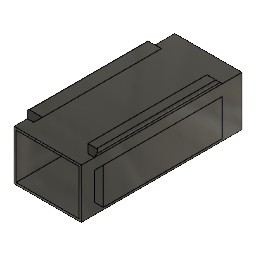
Res_Box v9 (Autodesk Fusion 360 design; units mm, degrees)
Autodesk Fusion 360 part; units mm, degrees
sketch "Boceto1" plane through (0, 0, 0) normal (0, 1, 0) x (1, 0, 0)
  line L0 (0, -22.6) -> (30.6, -22.6)
  line L1 (30.6, -22.6) -> (30.6, 0)
  line L2 (30.6, 0) -> (0, 0)
  line L3 (0, 0) -> (0, -22.6)
  dimension "d1" = 22.6
  dimension "d2" = 30.6
  constraint horizontal L0
  constraint vertical L1
  constraint horizontal L2
  constraint vertical L3
  constraint coincident L2.end L3.start
  measures "d1" distance of L0.end L1.end
  measures "d2" distance of L0.start L0.end
extrude "Extruir1" add sketch "Boceto1" along normal blind 73
shell "Vaciado1" thickness 1 removed faces 1 at (20.4, 0, 15.0667)
sketch "Boceto2" plane through (0, 0, 0) normal (0, -1, 0) x (1, 0, 0)
  line L0 (0, 22.6) -> (0, 0)
  line L1 (0, 0) -> (30.6, 0)
  line L2 (30.6, 0) -> (30.6, 22.6)
  line L3 (30.6, 22.6) -> (0, 22.6)
  line L4 (25.6, 24.6) -> (27.6, 22.6)
  line L5 (30.6, 23.6) -> (30.6, 22.6)
  line L6 (-2, 17.6) -> (-2, 22)
  line L7 (-2, 22) -> (-2, 23.6)
  line L8 (-1, 24.6) -> (0, 24.6)
  line L9 (-2, 17.6) -> (0, 19.6)
  line L10 (0, 24.6) -> (5, 24.6)
  line L11 (5, 24.6) -> (3, 22.6)
  line L12 (0, 0) -> (-1, 0)
  line L13 (-2, 1) -> (-2, 5)
  line L14 (-2, 5) -> (0, 3)
  line L15 (30.6, 17.6) -> (32.6, 19.6)
  line L16 (32.6, 19.6) -> (32.6, 3)
  line L17 (32.6, 3) -> (30.6, 5)
  line L18 (5, 0) -> (3, -2)
  line L19 (3, -2) -> (27.6, -2)
  line L20 (27.6, -2) -> (25.6, 0)
  line L21 (25.6, 24.6) -> (29.6, 24.6)
  line L22 (27.6, 22.6) -> (30.6, 22.6)
  line L23 (30.6, 17.6) -> (30.6, 5)
  line L24 (25.6, 0) -> (5, 0)
  line L25 (0, 0) -> (0, 3)
  line L26 (0, 19.6) -> (0, 22.6)
  arc A0 (-1, 24.6) -> (-2, 23.6) centre (-1, 23.6) ccw
  arc A1 (30.6, 23.6) -> (29.6, 24.6) centre (29.6, 23.6) ccw
  arc A2 (-2, 1) -> (-1, 0) centre (-1, 1) ccw
  line L27 (29.6, 1) -> (1, 1)
  line L28 (1, 1) -> (1, 21.6)
  line L29 (1, 21.6) -> (29.6, 21.6)
  line L30 (29.6, 21.6) -> (29.6, 1)
  dimension "d5" = 3
  dimension "d6" = 2
  dimension "d7" = 3
  dimension "d8" = 2
  dimension "d9" = 2
  dimension "d10" = 45
  dimension "d11" = 45
  dimension "d12" = 3
  dimension "d13" = 45
  dimension "d14" = 45
  dimension "d15" = 2
  dimension "d16" = 3
  dimension "d17" = 5
  dimension "d18" = 5
  dimension "d19" = 45
  dimension "d20" = 2
  dimension "d21" = 45
  dimension "d22" = 5
  dimension "d23" = 5
  dimension "d24" = 2
  dimension "d25" = 45
  dimension "d28" = 1
  dimension "d29" = 1
  dimension "d30" = 1
  constraint coincident L3 L4.end
  constraint coincident L2.end L3.start
  constraint parallel L0 L6
  constraint parallel L6 L7
  constraint perpendicular L7 L8
  constraint coincident L0 L9.end
  constraint parallel L8 L10
  constraint coincident L0.end L1.start
  constraint perpendicular L0 L12
  constraint perpendicular L12 L13
  constraint coincident L0 L14.end
  constraint coincident L2 L15.start
  constraint perpendicular L3 L16
  constraint coincident L2 L17.end
  constraint coincident L1 L18.start
  constraint perpendicular L14 L18
  constraint parallel L1 L19
  constraint coincident L1 L20.end
  constraint horizontal L21
  constraint coincident L0.start L3.end
  constraint coincident L3 L11.end
  constraint collinear L2 L5
  constraint tangent L7 A0
  constraint tangent L8 A0
  constraint tangent L5 A1
  constraint tangent L21 A1
  constraint tangent L12 A2
  constraint tangent L13 A2
  measures "d5" distance of L4.end L2.end
  measures "d6" distance of L3 L21
  measures "d7" distance of L0.start L11.end
  measures "d8" distance of L6 L26
  measures "d9" distance of L3 L10
  measures "d10" angle of L3 L11
  measures "d11" angle of L3 L4
  measures "d12" distance of L0.start L9.end
  measures "d13" angle of L0 L9
  measures "d14" angle of L0 L14
  measures "d15" distance of L0 L13
  measures "d16" distance of L0.end L14.end
  measures "d17" distance of L0.end L18.start
  measures "d18" distance of L1.end L20.end
  measures "d19" angle of L1 L20
  measures "d20" distance of L19 L24
  measures "d21" angle of L2 L17
  measures "d22" distance of L1.end L17.end
  measures "d23" distance of L2.end L15.start
  measures "d24" distance of L16 L23
  measures "d25" angle of L2 L15
  measures "d28" radius of A0
  measures "d29" radius of A1
  measures "d30" radius of A2
extrude "Extruir2" add sketch "Boceto2" against normal blind 64 contours L0 L3 L6 L7 L8 L9 L10 L11 L26 A0 | L0 L12 L13 L14 L25 A2 | L3 L4 L5 L21 L22 A1 | L1 L18 L19 L20 L24 | L2 L15 L16 L17 L23
sketch "Boceto3" plane through (0, 0, 0) normal (0, -1, 0) x (1, 0, 0)
  line L0 (29.6, 1) -> (1, 1)
  line L1 (1, 1) -> (1, 21.6)
  line L2 (1, 21.6) -> (29.6, 21.6)
  line L3 (29.6, 21.6) -> (29.6, 1)
  line L4 (-1, 0) -> (5, 0)
  line L5 (5, 0) -> (3, -2)
  line L6 (3, -2) -> (27.6, -2)
  line L7 (27.6, -2) -> (25.6, 0)
  line L8 (25.6, 0) -> (30.6, 0)
  line L9 (30.6, 0) -> (30.6, 5)
  line L10 (30.6, 5) -> (32.6, 3)
  line L11 (32.6, 3) -> (32.6, 19.6)
  line L12 (32.6, 19.6) -> (30.6, 17.6)
  line L13 (30.6, 17.6) -> (30.6, 22.6)
  line L14 (30.6, 22.6) -> (30.6, 23.6)
  arc A0 (30.6, 23.6) -> (29.6, 24.6) centre (29.6, 23.6) ccw
  line L15 (29.6, 24.6) -> (25.6, 24.6)
  line L16 (25.6, 24.6) -> (27.6, 22.6)
  line L17 (27.6, 22.6) -> (3, 22.6)
  line L18 (3, 22.6) -> (5, 24.6)
  line L19 (5, 24.6) -> (-1, 24.6)
  arc A1 (-1, 24.6) -> (-2, 23.6) centre (-1, 23.6) ccw
  line L20 (-2, 17.6) -> (0, 19.6)
  line L21 (0, 19.6) -> (0, 3)
  line L22 (0, 3) -> (-2, 5)
  line L23 (-2, 5) -> (-2, 1)
  arc A2 (-2, 1) -> (-1, 0) centre (-1, 1) ccw
  line L24 (0, 19.6) -> (-2, 17.6)
  line L25 (-1, 24.6) -> (5, 24.6)
  line L26 (3, 22.6) -> (0, 22.6)
  line L27 (0, 22.6) -> (0, 19.6)
  line L28 (27.6, 22.6) -> (25.6, 24.6)
  line L29 (30.6, 23.6) -> (30.6, 22.6)
  line L30 (27.6, 22.6) -> (30.6, 22.6)
  line L31 (32.6, 3) -> (30.6, 5)
  line L32 (30.6, 17.6) -> (32.6, 19.6)
  line L33 (30.6, 17.6) -> (30.6, 5)
  line L34 (-2, 23.6) -> (-2, 17.6)
  line L35 (32.6, 19.6) -> (32.6, 3)
  line L36 (27.6, -2) -> (25.6, 0)
  line L37 (5, 0) -> (3, -2)
  line L38 (27.6, -2) -> (3, -2)
  line L39 (5, 0) -> (25.6, 0)
  line L40 (-2, 1) -> (-2, 5)
  line L41 (0, 3) -> (0, 0)
  line L42 (-1, 0) -> (0, 0)
  arc A3 (-2, 1) -> (-1, 0) centre (-1, 1) ccw
  arc A4 (-1, 24.6) -> (-2, 23.6) centre (-1.0921, 23.6921) ccw
  line L43 (25.6, 24.6) -> (29.6, 24.6)
  arc A5 (30.6, 23.6) -> (29.6, 24.6) centre (29.6, 23.6) ccw
  arc A6 (-2, 1) -> (-1, 0) centre (-1, 1) ccw
  constraint coincident L20.end L21.start
  constraint coincident L20.start L24.end
  constraint coincident L19.end A1.start
  constraint coincident L18.end L19.start
  constraint coincident L17.end L18.start
  constraint parallel L17 L26
  constraint perpendicular L26 L27
  constraint coincident A1.end L34.start
  constraint coincident L16.end L17.start
  constraint coincident L15.end L16.start
  constraint coincident L14.end A0.start
  constraint coincident L13.end L14.start
  constraint coincident L10.end L11.start
  constraint coincident L9.end L10.start
  constraint coincident L12.end L13.start
  constraint coincident L11.end L12.start
  constraint coincident L6.end L7.start
  constraint coincident L7.end L8.start
  constraint coincident L4.end L5.start
  constraint coincident L5.end L6.start
  constraint coincident L23.end A2.start
  constraint coincident L22.end L23.start
  constraint coincident L21.end L22.start
  constraint coincident L41.end L42.end
  constraint coincident L4.start A2.end
  constraint coincident A0.end L15.start
  constraint tangent L14 A5
  constraint tangent L4 A6
extrude "Extruir3" cut sketch "Boceto3" against normal blind 6 contours L4 L22 L23 A2 L40 L41 L42 A3 A6 | L5 L6 L7 L36 L37 L38 L39 | L18 L19 A1 L20 L24 L25 L26 L27 L34 | L10 L11 L12 L31 L32 L33 L35 | L14 A0 L15 L16 L28 L29 L30 L43 A5
sketch "Boceto4" plane through (0, 73, 0) normal (0, 1, 0) x (-1, 0, 0)
  line L0 (0, 0) -> (0, 22.6)
  line L1 (0, 22.6) -> (-30.6, 22.6)
  line L2 (-30.6, 22.6) -> (-30.6, 0)
  line L3 (-30.6, 0) -> (0, 0)
  line L4 (-21.8, 17.3) -> (-8.8, 17.3)
  line L5 (-6.8, 15.3) -> (-6.8, 7.3)
  line L6 (-8.8, 5.3) -> (-21.8, 5.3)
  line L7 (-23.8, 7.3) -> (-23.8, 15.3)
  arc A0 (-21.8, 17.3) -> (-23.8, 15.3) centre (-21.8, 15.3) ccw
  arc A1 (-6.8, 15.3) -> (-8.8, 17.3) centre (-8.8, 15.3) ccw
  arc A2 (-8.8, 5.3) -> (-6.8, 7.3) centre (-8.8, 7.3) ccw
  arc A3 (-23.8, 7.3) -> (-21.8, 5.3) centre (-21.8, 7.3) ccw
  line L8 (-15.3, 17.3) -> (-15.3, 5.3) construction
  line L9 (-23.8, 11.3) -> (-6.8, 11.3) construction
  point P0 (-23.8, 17.3)
  point P1 (-6.8, 17.3)
  point P2 (-6.8, 5.3)
  dimension "d44" = 2
  dimension "d45" = 2
  dimension "d46" = 2
  dimension "d47" = 2
  dimension "d48" = 17
  dimension "d50" = 15.3
  dimension "d51" = 12
  dimension "d52" = 11.3
  constraint horizontal L4
  constraint vertical L5
  constraint horizontal L6
  constraint vertical L7
  constraint coincident P0 L4
  constraint coincident P0 L7
  constraint tangent L4 A0
  constraint tangent L7 A0
  constraint coincident P1 L4
  constraint coincident P1 L5
  constraint tangent L4 A1
  constraint tangent L5 A1
  constraint coincident P2 L5
  constraint coincident P2 L6
  constraint tangent L5 A2
  constraint tangent L6 A2
  constraint tangent L7 A3
  constraint tangent L6 A3
  constraint midpoint L4 L8.start
  constraint midpoint L6 L8.end
  constraint midpoint L7 L9.start
  constraint midpoint L5 L9.end
  measures "d44" radius of A0
  measures "d45" radius of A1
  measures "d46" radius of A2
  measures "d47" radius of A3
  measures "d48" distance of L5 L7
  measures "d50" distance of L2 L8
  measures "d51" distance of L4 L6
  measures "d52" distance of L3 L9
extrude "Extruir4" cut sketch "Boceto4" against normal blind 1 contours L4 L5 L6 L7 A0 A1 A2 A3
chamfer "Chaflán2" distance 2 angle 45 4 edges at (32.6, 6, 11.3) (15.3, 6, -2) (32.6, 64, 11.3) (15.3, 64, -2)
sketch "Boceto5" plane through (30.6, 0, 0) normal (1, 0, 0) x (0, 1, 0)
  line L0 (6, 23.6) -> (6, 22.6)
  line L1 (6, 22.6) -> (64, 22.6)
  line L2 (64, 22.6) -> (64, 23.6)
  line L3 (64, 23.6) -> (6, 23.6)
  line L4 (6, 22.6) -> (6, 24.6)
  line L5 (6, 24.6) -> (8, 24.6)
  line L6 (8, 24.6) -> (6, 22.6)
  line L7 (64, 22.6) -> (64, 24.6)
  line L8 (64, 24.6) -> (62, 24.6)
  line L9 (62, 24.6) -> (64, 22.6)
  dimension "d54" = 2
  dimension "d55" = 45
  dimension "d58" = 2
  dimension "d59" = 45
  constraint coincident L0.end L1.start
  constraint perpendicular L3 L4
  constraint perpendicular L4 L5
  constraint perpendicular L7 L8
  constraint coincident L1.end L2.start
  constraint collinear L2 L7
  measures "d54" distance of L4.end L5.end
  measures "d55" angle of L1 L6
  measures "d58" distance of L7.end L8.end
  measures "d59" angle of L1 L9
extrude "Extruir5" cut sketch "Boceto5" against normal blind 33 contours L0 L3 L4 L6 | L3 L4 L5 L6 | L2 L3 L7 L9 | L3 L7 L8 L9
sketch "Boceto6" plane through (0, 0, 0) normal (0, 0, -1) x (1, 0, 0)
  line L0 (30.6, 0) -> (0, 0)
  line L1 (0, 0) -> (0, -6)
  line L2 (0, -6) -> (-1, -6)
  line L3 (-1, -6) -> (-1, -64)
  line L4 (-1, -64) -> (0, -64)
  line L5 (0, -64) -> (0, -73)
  line L6 (0, -73) -> (30.6, -73)
  line L7 (30.6, -73) -> (30.6, 0)
  line L8 (5, -6) -> (25.6, -6)
  line L9 (25.6, -6) -> (25.6, -64)
  line L10 (25.6, -64) -> (5, -64)
  line L11 (5, -64) -> (5, -6)
  line L12 (0, -6) -> (-2, -8)
  line L13 (-2, -8) -> (-2, -6)
  line L14 (-2, -6) -> (0, -6)
  line L15 (0, -64) -> (-2, -64)
  line L16 (-2, -64) -> (-2, -62)
  line L17 (-2, -62) -> (0, -64)
  dimension "d60" = 2
  dimension "d61" = 45
  dimension "d62" = 45
  dimension "d63" = 2
  constraint coincident L1.end L2.start
  constraint perpendicular L2 L13
  constraint perpendicular L1 L14
  constraint coincident L4.end L5.start
  constraint perpendicular L3 L15
  constraint perpendicular L4 L16
  measures "d60" distance of L12.end L13.end
  measures "d61" angle of L1 L12
  measures "d62" angle of L5 L17
  measures "d63" distance of L15.end L16.end
extrude "Extruir6" cut sketch "Boceto6" against normal blind 24.8 contours L2 L3 L12 L14 | L3 L12 L13 L14 | L3 L4 L15 L17 | L3 L15 L16 L17
sketch "Boceto7" plane through (0, 0, 21.6) normal (0, 0, -1) x (1, 0, 0)
  line L0 (29.6, 0) -> (1, 0)
  line L1 (1, 0) -> (1, -72)
  line L2 (1, -72) -> (29.6, -72)
  line L3 (29.6, -72) -> (29.6, 0)
  line L4 (4.3, -1) -> (26.3, -1)
  line L5 (26.3, -1) -> (26.3, -3)
  line L6 (26.3, -3) -> (4.3, -3)
  line L7 (4.3, -3) -> (4.3, -1)
  line L8 (15.3, -1) -> (15.3, -3) construction
  line L9 (0, 0) -> (0, -6)
  dimension "d66" = 1
  dimension "d67" = 22
  dimension "d68" = 2
  dimension "d69" = 15.3
  constraint horizontal L4
  constraint vertical L5
  constraint horizontal L6
  constraint vertical L7
  constraint midpoint L4 L8.start
  constraint midpoint L6 L8.end
  measures "d66" distance of L0 L4
  measures "d67" distance of L5.end L6.end
  measures "d68" distance of L4.end L5.end
  measures "d69" distance of L8 L9
extrude "Extruir7" add sketch "Boceto7" along normal blind 1 contours L4 L5 L6 L7
sketch "Boceto8" plane through (0, 0, 20.6) normal (0, 0, -1) x (1, 0, 0)
  line L0 (4.3, -3) -> (26.3, -3)
  line L1 (26.3, -3) -> (26.3, -1)
  line L2 (26.3, -1) -> (4.3, -1)
  line L3 (4.3, -1) -> (4.3, -3)
  line L4 (4.3, -1) -> (6.3, -1)
  line L5 (6.3, -1) -> (6.3, -3)
  line L6 (6.3, -3) -> (4.3, -3)
  line L7 (4.3, -3) -> (4.3, -1)
  line L8 (26.3, -3) -> (24.3, -3)
  line L9 (24.3, -3) -> (24.3, -1)
  line L10 (24.3, -1) -> (26.3, -1)
  line L11 (26.3, -1) -> (26.3, -3)
  dimension "d72" = 2
  dimension "d73" = 2
  constraint horizontal L4
  constraint vertical L5
  constraint horizontal L6
  constraint vertical L7
  constraint coincident L0 L5.end
  constraint coincident L2.end L3.start
  constraint horizontal L8
  constraint vertical L9
  constraint horizontal L10
  constraint vertical L11
  constraint coincident L2 L9.end
  constraint coincident L0.end L1.start
  measures "d72" distance of L2.end L4.end
  measures "d73" distance of L9.end L1.end
extrude "Extruir8" add sketch "Boceto8" along normal blind 1 contours L0 L2 L3 L4 L5 L6 L7 | L0 L1 L2 L8 L9 L10 L11
chamfer "Chaflán3" distance 1 angle 45 2 edges at (5.3, 1, 19.6) (25.3, 1, 19.6)
equation "d1 = external_heigth"
equation "d2 = external_width"
equation "d3 = external_depth + 1 mm"
equation "external_width = 30.6 mm"
equation "external_heigth = 22.6 mm"
equation "external_depth = 72 mm"
equation "d50 = external_width / 2"
equation "d52 = external_heigth / 2"
equation "d69 = external_width / 2"
